Autodesk Fusion 360 part; units mm, degrees
note: some values were not read from the file. Set by a fixed rule: which sketch regions a step uses.
(part 19 of 20)
  spline S109 degree 5 poles (-22.9448, 17.8091) (-22.9448, 17.8092) (-22.945, 17.8093) (-22.9453, 17.8095) (-22.9457, 17.8098) (-22.9463, 17.8103) (-22.9469, 17.8108) (-22.9477, 17.8114) (-22.9486, 17.812) (-22.9496, 17.8127) (-22.9506, 17.8135) (-22.9518, 17.8144) (-22.953, 17.8153) (-22.9543, 17.8162) (-22.9557, 17.8172) (-22.9572, 17.8183) (-22.9588, 17.8195) (-22.9604, 17.8207) (-22.9622, 17.8219) (-22.964, 17.8232) (-22.9659, 17.8246) (-22.9679, 17.826) (-22.9699, 17.8274) (-22.9721, 17.8289) (-22.9743, 17.8305) (-22.9766, 17.8321) (-22.979, 17.8337) (-22.9814, 17.8354) (-22.984, 17.8372) (-22.9866, 17.8389) (-22.9893, 17.8408) (-22.992, 17.8427) (-22.9948, 17.8446) (-22.9978, 17.8465) (-23.0007, 17.8485) (-23.0038, 17.8506) (-23.0069, 17.8527) (-23.0101, 17.8548) (-23.0134, 17.857) (-23.0167, 17.8592) (-23.0201, 17.8614) (-23.0236, 17.8637) (-23.0271, 17.866) (-23.0308, 17.8683) (-23.0344, 17.8707) (-23.0382, 17.8731) (-23.042, 17.8756) (-23.0459, 17.8781) (-23.0499, 17.8806) (-23.0539, 17.8831) (-23.058, 17.8857) (-23.0621, 17.8883) (-23.0664, 17.891) (-23.0706, 17.8937) (-23.075, 17.8964) (-23.0794, 17.8991) (-23.0839, 17.9019) (-23.0884, 17.9047) (-23.093, 17.9075) (-23.0977, 17.9103) (-23.1024, 17.9132) (-23.1072, 17.9161) (-23.1121, 17.9191) (-23.117, 17.922) (-23.122, 17.925) (-23.127, 17.928) (-23.1321, 17.931) (-23.1373, 17.9341) (-23.1425, 17.9372) (-23.1478, 17.9403) (-23.1531, 17.9434) (-23.1585, 17.9466) (-23.164, 17.9497) (-23.1695, 17.9529) (-23.1751, 17.9562) (-23.1807, 17.9594) (-23.1864, 17.9627) (-23.1921, 17.9659) (-23.1979, 17.9692) (-23.2038, 17.9726) (-23.2097, 17.9759) (-23.2157, 17.9793) (-23.2217, 17.9826) (-23.2278, 17.986) (-23.234, 17.9895) (-23.2402, 17.9929) (-23.2464, 17.9963) (-23.2527, 17.9998) (-23.2591, 18.0033) (-23.2655, 18.0068) (-23.272, 18.0103) (-23.2785, 18.0139) (-23.2851, 18.0174) (-23.2918, 18.021) (-23.2984, 18.0246) (-23.3052, 18.0282) (-23.312, 18.0318) (-23.3188, 18.0354) (-23.3257, 18.039) (-23.3327, 18.0427) (-23.3397, 18.0464) (-23.3468, 18.0501) (-23.3539, 18.0538) (-23.361, 18.0575) (-23.3683, 18.0612) (-23.3755, 18.0649) (-23.3828, 18.0687) (-23.3902, 18.0724) (-23.3976, 18.0762) (-23.4051, 18.08) (-23.4126, 18.0838) (-23.4202, 18.0876) (-23.4278, 18.0914) (-23.4355, 18.0952) (-23.4432, 18.0991) (-23.451, 18.1029) (-23.4588, 18.1068) (-23.4666, 18.1106) (-23.4746, 18.1145) (-23.4825, 18.1184) (-23.4905, 18.1223) (-23.4986, 18.1262) (-23.5067, 18.1301) (-23.5149, 18.134) (-23.5231, 18.1379) (-23.5313, 18.1419) (-23.5396, 18.1458) (-23.548, 18.1498) (-23.5564, 18.1537) (-23.5648, 18.1577) (-23.5733, 18.1617) (-23.5818, 18.1657) (-23.5904, 18.1696) (-23.5991, 18.1736) (-23.6077, 18.1776) (-23.6165, 18.1816) (-23.6252, 18.1857) (-23.634, 18.1897) (-23.6429, 18.1937) (-23.6518, 18.1977) (-23.6607, 18.2018) (-23.6697, 18.2058) (-23.6788, 18.2098) (-23.6879, 18.2139) (-23.697, 18.2179) (-23.7062, 18.222) (-23.7154, 18.226) (-23.7247, 18.2301) (-23.734, 18.2342) (-23.7433, 18.2383) (-23.7527, 18.2423) (-23.7622, 18.2464) (-23.7716, 18.2505) (-23.7812, 18.2546) (-23.7907, 18.2587) (-23.8004, 18.2627) (-23.81, 18.2668) (-23.8197, 18.2709) (-23.8295, 18.275) (-23.8393, 18.2791) (-23.8491, 18.2832) (-23.859, 18.2873) (-23.8689, 18.2914) (-23.8788, 18.2955) (-23.8888, 18.2996) (-23.8989, 18.3038) (-23.909, 18.3079) (-23.9191, 18.312) (-23.9292, 18.3161) (-23.9395, 18.3202) (-23.9497, 18.3243) (-23.96, 18.3284) (-23.9703, 18.3325) (-23.9807, 18.3366) (-23.9911, 18.3408) (-24.0016, 18.3449) (-24.0121, 18.349) (-24.0226, 18.3531) (-24.0332, 18.3572) (-24.0438, 18.3613) (-24.0545, 18.3654) (-24.0652, 18.3695) (-24.0759, 18.3736) (-24.0867, 18.3777) (-24.0975, 18.3818) (-24.1084, 18.3859) (-24.1193, 18.39) (-24.1302, 18.3941) (-24.1412, 18.3982) (-24.1522, 18.4023) (-24.1633, 18.4064) (-24.1744, 18.4105) (-24.1855, 18.4146) (-24.1967, 18.4187) (-24.2079, 18.4228) (-24.2191, 18.4269) (-24.2304, 18.4309) (-24.2417, 18.435) (-24.2531, 18.4391) (-24.2645, 18.4431) (-24.276, 18.4472) (-24.2874, 18.4513) (-24.299, 18.4553) (-24.3105, 18.4594) (-24.3221, 18.4634) (-24.3337, 18.4675) (-24.3454, 18.4715) (-24.3571, 18.4756) (-24.3689, 18.4796) (-24.3806, 18.4836) (-24.3925, 18.4877) (-24.4043, 18.4917) (-24.4162, 18.4957) (-24.4281, 18.4997) (-24.4401, 18.5037) (-24.4521, 18.5077) (-24.4642, 18.5117) (-24.4762, 18.5157) (-24.4884, 18.5197) (-24.5005, 18.5237) (-24.5127, 18.5277) (-24.5249, 18.5316) (-24.5372, 18.5356) (-24.5495, 18.5395) (-24.5618, 18.5435) (-24.5742, 18.5475) (-24.5866, 18.5514) (-24.599, 18.5553) (-24.6115, 18.5593) (-24.624, 18.5632) (-24.6365, 18.5671) (-24.6491, 18.571) (-24.6617, 18.5749) (-24.6744, 18.5788) (-24.6871, 18.5827) (-24.6998, 18.5866) (-24.7125, 18.5905) (-24.7253, 18.5943) (-24.7382, 18.5982) (-24.751, 18.6021) (-24.7639, 18.6059) (-24.7743, 18.609) (-24.782, 18.6113) (-24.7872, 18.6128) (-24.7898, 18.6136) knots 0 0 0 0 0 0 0.00416667 0.00833333 0.0125 0.01666667 0.02083333 0.025 0.02916667 0.03333333 0.0375 0.04166667 0.04583333 0.05 0.05416667 0.05833333 0.0625 0.06666667 0.07083333 0.075 0.07916667 0.08333333 0.0875 0.09166667 0.09583333 0.1 0.10416667 0.10833333 0.1125 0.11666667 0.12083333 0.125 0.12916667 0.13333333 0.1375 0.14166667 0.14583333 0.15 0.15416667 0.15833333 0.1625 0.16666667 0.17083333 0.175 0.17916667 0.18333333 0.1875 0.19166667 0.19583333 0.2 0.20416667 0.20833333 0.2125 0.21666667 0.22083333 0.225 0.22916667 0.23333333 0.2375 0.24166667 0.24583333 0.25 0.25416667 0.25833333 0.2625 0.26666667 0.27083333 0.275 0.27916667 0.28333333 0.2875 0.29166667 0.29583333 0.3 0.30416667 0.30833333 0.3125 0.31666667 0.32083333 0.325 0.32916667 0.33333333 0.3375 0.34166667 0.34583333 0.35 0.35416667 0.35833333 0.3625 0.36666667 0.37083333 0.375 0.37916667 0.38333333 0.3875 0.39166667 0.39583333 0.4 0.40416667 0.40833333 0.4125 0.41666667 0.42083333 0.425 0.42916667 0.43333333 0.4375 0.44166667 0.44583333 0.45 0.45416667 0.45833333 0.4625 0.46666667 0.47083333 0.475 0.47916667 0.48333333 0.4875 0.49166667 0.49583333 0.5 0.50416667 0.50833333 0.5125 0.51666667 0.52083333 0.525 0.52916667 0.53333333 0.5375 0.54166667 0.54583333 0.55 0.55416667 0.55833333 0.5625 0.56666667 0.57083333 0.575 0.57916667 0.58333333 0.5875 0.59166667 0.59583333 0.6 0.60416667 0.60833333 0.6125 0.61666667 0.62083333 0.625 0.62916667 0.63333333 0.6375 0.64166667 0.64583333 0.65 0.65416667 0.65833333 0.6625 0.66666667 0.67083333 0.675 0.67916667 0.68333333 0.6875 0.69166667 0.69583333 0.7 0.70416667 0.70833333 0.7125 0.71666667 0.72083333 0.725 0.72916667 0.73333333 0.7375 0.74166667 0.74583333 0.75 0.75416667 0.75833333 0.7625 0.76666667 0.77083333 0.775 0.77916667 0.78333333 0.7875 0.79166667 0.79583333 0.8 0.80416667 0.80833333 0.8125 0.81666667 0.82083333 0.825 0.82916667 0.83333333 0.8375 0.84166667 0.84583333 0.85 0.85416667 0.85833333 0.8625 0.86666667 0.87083333 0.875 0.87916667 0.88333333 0.8875 0.89166667 0.89583333 0.9 0.90416667 0.90833333 0.9125 0.91666667 0.92083333 0.925 0.92916667 0.93333333 0.9375 0.94166667 0.94583333 0.95 0.95416667 0.95833333 0.9625 0.96666667 0.97083333 0.975 0.97916667 0.98333333 0.9875 0.99166667 0.99583333 1 1 1 1 1 1
  line L217 (-20.9569, 20.1094) -> (-20.9575, 20.11)
  line L218 (-13.7175, -25.6019) -> (-13.7171, -25.6012)
  line L219 (-10.9659, -26.8948) -> (-10.8547, -26.6221)
  arc A111 (30.4202, 5.9675) -> (30.2174, 6.9214) centre (0, 0) ccw
  arc A112 (27.918, 6.8665) -> (27.6109, 8.0125) centre (0, 0) ccw
  line L220 (-24.0278, 16.3184) -> (-24.0271, 16.318)
  spline S110 degree 5 poles (3.9508, 28.7753) (3.9508, 28.7754) (3.9508, 28.7756) (3.9509, 28.7759) (3.9509, 28.7764) (3.951, 28.7772) (3.9511, 28.778) (3.9512, 28.779) (3.9514, 28.7801) (3.9515, 28.7813) (3.9517, 28.7826) (3.9518, 28.784) (3.952, 28.7855) (3.9522, 28.7871) (3.9523, 28.7889) (3.9525, 28.7907) (3.9527, 28.7926) (3.9529, 28.7946) (3.9531, 28.7968) (3.9534, 28.799) (3.9536, 28.8013) (3.9538, 28.8037) (3.954, 28.8063) (3.9543, 28.8089) (3.9545, 28.8116) (3.9547, 28.8144) (3.955, 28.8172) (3.9552, 28.8202) (3.9555, 28.8233) (3.9557, 28.8264) (3.9559, 28.8297) (3.9562, 28.833) (3.9564, 28.8364) (3.9567, 28.8399) (3.9569, 28.8435) (3.9572, 28.8472) (3.9574, 28.8509) (3.9577, 28.8547) (3.9579, 28.8586) (3.9581, 28.8626) (3.9584, 28.8667) (3.9586, 28.8709) (3.9588, 28.8751) (3.959, 28.8794) (3.9593, 28.8838) (3.9595, 28.8882) (3.9597, 28.8928) (3.9599, 28.8974) (3.9601, 28.9021) (3.9603, 28.9068) (3.9605, 28.9117) (3.9607, 28.9166) (3.9609, 28.9215) (3.961, 28.9266) (3.9612, 28.9317) (3.9614, 28.9369) (3.9615, 28.9422) (3.9617, 28.9475) (3.9618, 28.9529) (3.962, 28.9584) (3.9621, 28.9639) (3.9622, 28.9695) (3.9623, 28.9752) (3.9624, 28.9809) (3.9625, 28.9867) (3.9626, 28.9926) (3.9627, 28.9985) (3.9627, 29.0045) (3.9628, 29.0106) (3.9629, 29.0167) (3.9629, 29.0229) (3.9629, 29.0291) (3.9629, 29.0355) (3.963, 29.0418) (3.963, 29.0483) (3.9629, 29.0548) (3.9629, 29.0613) (3.9629, 29.068) (3.9628, 29.0746) (3.9628, 29.0814) (3.9627, 29.0882) (3.9626, 29.095) (3.9626, 29.1019) (3.9625, 29.1089) (3.9623, 29.1159) (3.9622, 29.123) (3.9621, 29.1302) (3.9619, 29.1374) (3.9618, 29.1446) (3.9616, 29.1519) (3.9614, 29.1593) (3.9612, 29.1667) (3.961, 29.1742) (3.9607, 29.1817) (3.9605, 29.1893) (3.9603, 29.197) (3.96, 29.2047) (3.9597, 29.2124) (3.9594, 29.2202) (3.9591, 29.2281) (3.9588, 29.236) (3.9584, 29.2439) (3.9581, 29.2519) (3.9577, 29.26) (3.9573, 29.2681) (3.9569, 29.2763) (3.9565, 29.2845) (3.9561, 29.2927) (3.9556, 29.301) (3.9552, 29.3094) (3.9547, 29.3178) (3.9542, 29.3263) (3.9537, 29.3348) (3.9532, 29.3433) (3.9526, 29.3519) (3.9521, 29.3606) (3.9515, 29.3693) (3.9509, 29.378) (3.9503, 29.3868) (3.9497, 29.3957) (3.9491, 29.4045) (3.9484, 29.4135) (3.9478, 29.4225) (3.9471, 29.4315) (3.9464, 29.4406) (3.9457, 29.4497) (3.9449, 29.4588) (3.9442, 29.468) (3.9434, 29.4773) (3.9426, 29.4866) (3.9418, 29.4959) (3.941, 29.5053) (3.9402, 29.5147) (3.9393, 29.5242) (3.9384, 29.5337) (3.9375, 29.5433) (3.9366, 29.5529) (3.9357, 29.5625) (3.9348, 29.5722) (3.9338, 29.5819) (3.9328, 29.5917) (3.9318, 29.6015) (3.9308, 29.6113) (3.9297, 29.6212) (3.9287, 29.6312) (3.9276, 29.6411) (3.9265, 29.6512) (3.9254, 29.6612) (3.9243, 29.6713) (3.9231, 29.6814) (3.922, 29.6916) (3.9208, 29.7018) (3.9196, 29.7121) (3.9183, 29.7224) (3.9171, 29.7327) (3.9158, 29.7431) (3.9145, 29.7535) (3.9132, 29.764) (3.9119, 29.7744) (3.9106, 29.785) (3.9092, 29.7955) (3.9078, 29.8061) (3.9064, 29.8168) (3.905, 29.8274) (3.9035, 29.8382) (3.9021, 29.8489) (3.9006, 29.8597) (3.8991, 29.8705) (3.8976, 29.8814) (3.896, 29.8923) (3.8945, 29.9032) (3.8929, 29.9142) (3.8913, 29.9252) (3.8896, 29.9362) (3.888, 29.9473) (3.8863, 29.9584) (3.8846, 29.9696) (3.8829, 29.9807) (3.8812, 29.992) (3.8795, 30.0032) (3.8777, 30.0145) (3.8759, 30.0258) (3.8741, 30.0372) (3.8722, 30.0486) (3.8704, 30.06) (3.8685, 30.0714) (3.8666, 30.0829) (3.8647, 30.0944) (3.8628, 30.106) (3.8608, 30.1176) (3.8588, 30.1292) (3.8568, 30.1409) (3.8548, 30.1525) (3.8527, 30.1643) (3.8507, 30.176) (3.8486, 30.1878) (3.8464, 30.1996) (3.8443, 30.2115) (3.8422, 30.2233) (3.84, 30.2353) (3.8378, 30.2472) (3.8356, 30.2592) (3.8333, 30.2712) (3.831, 30.2832) (3.8288, 30.2953) (3.8264, 30.3074) (3.8241, 30.3195) (3.8217, 30.3317) (3.8194, 30.3439) (3.817, 30.3561) (3.8145, 30.3683) (3.8121, 30.3806) (3.8096, 30.3929) (3.8071, 30.4053) (3.8046, 30.4176) (3.8021, 30.43) (3.7995, 30.4424) (3.797, 30.4549) (3.7943, 30.4674) (3.7917, 30.4799) (3.7891, 30.4924) (3.7864, 30.505) (3.7837, 30.5176) (3.781, 30.5302) (3.7782, 30.5429) (3.7755, 30.5556) (3.7727, 30.5683) (3.7699, 30.581) (3.767, 30.5938) (3.7642, 30.6066) (3.7613, 30.6194) (3.7584, 30.6323) (3.7555, 30.6451) (3.7525, 30.658) (3.7496, 30.671) (3.7466, 30.6839) (3.7435, 30.6969) (3.7405, 30.7099) (3.7374, 30.723) (3.7343, 30.736) (3.7312, 30.7491) (3.7287, 30.7596) (3.7268, 30.7675) (3.7256, 30.7728) (3.7249, 30.7754) knots 0 0 0 0 0 0 0.00416667 0.00833333 0.0125 0.01666667 0.02083333 0.025 0.02916667 0.03333333 0.0375 0.04166667 0.04583333 0.05 0.05416667 0.05833333 0.0625 0.06666667 0.07083333 0.075 0.07916667 0.08333333 0.0875 0.09166667 0.09583333 0.1 0.10416667 0.10833333 0.1125 0.11666667 0.12083333 0.125 0.12916667 0.13333333 0.1375 0.14166667 0.14583333 0.15 0.15416667 0.15833333 0.1625 0.16666667 0.17083333 0.175 0.17916667 0.18333333 0.1875 0.19166667 0.19583333 0.2 0.20416667 0.20833333 0.2125 0.21666667 0.22083333 0.225 0.22916667 0.23333333 0.2375 0.24166667 0.24583333 0.25 0.25416667 0.25833333 0.2625 0.26666667 0.27083333 0.275 0.27916667 0.28333333 0.2875 0.29166667 0.29583333 0.3 0.30416667 0.30833333 0.3125 0.31666667 0.32083333 0.325 0.32916667 0.33333333 0.3375 0.34166667 0.34583333 0.35 0.35416667 0.35833333 0.3625 0.36666667 0.37083333 0.375 0.37916667 0.38333333 0.3875 0.39166667 0.39583333 0.4 0.40416667 0.40833333 0.4125 0.41666667 0.42083333 0.425 0.42916667 0.43333333 0.4375 0.44166667 0.44583333 0.45 0.45416667 0.45833333 0.4625 0.46666667 0.47083333 0.475 0.47916667 0.48333333 0.4875 0.49166667 0.49583333 0.5 0.50416667 0.50833333 0.5125 0.51666667 0.52083333 0.525 0.52916667 0.53333333 0.5375 0.54166667 0.54583333 0.55 0.55416667 0.55833333 0.5625 0.56666667 0.57083333 0.575 0.57916667 0.58333333 0.5875 0.59166667 0.59583333 0.6 0.60416667 0.60833333 0.6125 0.61666667 0.62083333 0.625 0.62916667 0.63333333 0.6375 0.64166667 0.64583333 0.65 0.65416667 0.65833333 0.6625 0.66666667 0.67083333 0.675 0.67916667 0.68333333 0.6875 0.69166667 0.69583333 0.7 0.70416667 0.70833333 0.7125 0.71666667 0.72083333 0.725 0.72916667 0.73333333 0.7375 0.74166667 0.74583333 0.75 0.75416667 0.75833333 0.7625 0.76666667 0.77083333 0.775 0.77916667 0.78333333 0.7875 0.79166667 0.79583333 0.8 0.80416667 0.80833333 0.8125 0.81666667 0.82083333 0.825 0.82916667 0.83333333 0.8375 0.84166667 0.84583333 0.85 0.85416667 0.85833333 0.8625 0.86666667 0.87083333 0.875 0.87916667 0.88333333 0.8875 0.89166667 0.89583333 0.9 0.90416667 0.90833333 0.9125 0.91666667 0.92083333 0.925 0.92916667 0.93333333 0.9375 0.94166667 0.94583333 0.95 0.95416667 0.95833333 0.9625 0.96666667 0.97083333 0.975 0.97916667 0.98333333 0.9875 0.99166667 0.99583333 1 1 1 1 1 1
  arc A113 (3.7249, 30.7754) -> (2.755, 30.8773) centre (0, 0) ccw
  circle A114 centre (0, 10) radius 1.7
  spline S111 degree 5 poles (-27.0873, 15.0758) (-27.0855, 15.0737) (-27.082, 15.0696) (-27.0767, 15.0635) (-27.0697, 15.0553) (-27.061, 15.045) (-27.0522, 15.0349) (-27.0435, 15.0247) (-27.0347, 15.0146) (-27.026, 15.0045) (-27.0173, 14.9945) (-27.0086, 14.9845) (-26.9999, 14.9745) (-26.9912, 14.9646) (-26.9825, 14.9547) (-26.9738, 14.9448) (-26.9651, 14.935) (-26.9565, 14.9252) (-26.9478, 14.9154) (-26.9392, 14.9057) (-26.9305, 14.896) (-26.9219, 14.8863) (-26.9133, 14.8767) (-26.9047, 14.8671) (-26.8961, 14.8576) (-26.8875, 14.8481) (-26.8789, 14.8386) (-26.8703, 14.8291) (-26.8618, 14.8197) (-26.8532, 14.8104) (-26.8447, 14.801) (-26.8361, 14.7917) (-26.8276, 14.7824) (-26.8191, 14.7732) (-26.8106, 14.764) (-26.8021, 14.7549) (-26.7937, 14.7457) (-26.7852, 14.7366) (-26.7767, 14.7276) (-26.7683, 14.7186) (-26.7599, 14.7096) (-26.7515, 14.7006) (-26.7431, 14.6917) (-26.7347, 14.6829) (-26.7263, 14.674) (-26.7179, 14.6652) (-26.7096, 14.6565) (-26.7012, 14.6477) (-26.6929, 14.639) (-26.6846, 14.6304) (-26.6763, 14.6218) (-26.668, 14.6132) (-26.6597, 14.6046) (-26.6514, 14.5961) (-26.6432, 14.5877) (-26.635, 14.5792) (-26.6267, 14.5708) (-26.6185, 14.5625) (-26.6103, 14.5541) (-26.6022, 14.5459) (-26.594, 14.5376) (-26.5858, 14.5294) (-26.5777, 14.5212) (-26.5696, 14.5131) (-26.5615, 14.505) (-26.5534, 14.4969) (-26.5453, 14.4889) (-26.5373, 14.4809) (-26.5292, 14.4729) (-26.5212, 14.465) (-26.5132, 14.4571) (-26.5052, 14.4493) (-26.4972, 14.4415) (-26.4893, 14.4337) (-26.4813, 14.426) (-26.4734, 14.4183) (-26.4655, 14.4106) (-26.4576, 14.403) (-26.4497, 14.3954) (-26.4419, 14.3879) (-26.434, 14.3804) (-26.4262, 14.3729) (-26.4184, 14.3655) (-26.4106, 14.3581) (-26.4029, 14.3508) (-26.3951, 14.3435) (-26.3874, 14.3362) (-26.3797, 14.3289) (-26.372, 14.3217) (-26.3643, 14.3146) (-26.3567, 14.3075) (-26.3491, 14.3004) (-26.3414, 14.2933) (-26.3339, 14.2863) (-26.3263, 14.2794) (-26.3188, 14.2724) (-26.3112, 14.2656) (-26.3037, 14.2587) (-26.2962, 14.2519) (-26.2888, 14.2451) (-26.2813, 14.2384) (-26.2739, 14.2317) (-26.2665, 14.225) (-26.2592, 14.2184) (-26.2518, 14.2119) (-26.2445, 14.2053) (-26.2372, 14.1988) (-26.2299, 14.1924) (-26.2227, 14.1859) (-26.2154, 14.1796) (-26.2082, 14.1732) (-26.201, 14.1669) (-26.1939, 14.1607) (-26.1868, 14.1544) (-26.1796, 14.1483) (-26.1726, 14.1421) (-26.1655, 14.136) (-26.1585, 14.13) (-26.1515, 14.1239) (-26.1445, 14.118) (-26.1375, 14.112) (-26.1306, 14.1061) (-26.1237, 14.1003) (-26.1168, 14.0945) (-26.11, 14.0887) (-26.1032, 14.0829) (-26.0964, 14.0772) (-26.0896, 14.0716) (-26.0829, 14.066) (-26.0762, 14.0604) (-26.0695, 14.0549) (-26.0629, 14.0494) (-26.0563, 14.0439) (-26.0497, 14.0385) (-26.0431, 14.0332) (-26.0366, 14.0278) (-26.0301, 14.0225) (-26.0236, 14.0173) (-26.0172, 14.0121) (-26.0108, 14.0069) (-26.0044, 14.0018) (-25.9981, 13.9967) (-25.9918, 13.9917) (-25.9855, 13.9867) (-25.9793, 13.9818) (-25.9731, 13.9769) (-25.9669, 13.972) (-25.9608, 13.9672) (-25.9547, 13.9624) (-25.9486, 13.9576) (-25.9426, 13.9529) (-25.9366, 13.9483) (-25.9306, 13.9437) (-25.9247, 13.9391) (-25.9188, 13.9346) (-25.913, 13.9301) (-25.9072, 13.9257) (-25.9014, 13.9213) (-25.8957, 13.9169) (-25.89, 13.9126) (-25.8843, 13.9083) (-25.8787, 13.9041) (-25.8731, 13.8999) (-25.8676, 13.8958) (-25.8621, 13.8917) (-25.8566, 13.8876) (-25.8512, 13.8836) (-25.8458, 13.8797) (-25.8405, 13.8758) (-25.8352, 13.8719) (-25.8299, 13.8681) (-25.8247, 13.8643) (-25.8195, 13.8605) (-25.8144, 13.8568) (-25.8093, 13.8532) (-25.8043, 13.8496) (-25.7993, 13.846) (-25.7944, 13.8425) (-25.7895, 13.839) (-25.7847, 13.8356) (-25.7799, 13.8322) (-25.7751, 13.8289) (-25.7704, 13.8256) (-25.7658, 13.8224) (-25.7612, 13.8192) (-25.7566, 13.816) (-25.7521, 13.8129) (-25.7476, 13.8098) (-25.7432, 13.8068) (-25.7389, 13.8039) (-25.7346, 13.8009) (-25.7304, 13.7981) (-25.7262, 13.7952) (-25.722, 13.7925) (-25.718, 13.7897) (-25.7139, 13.787) (-25.71, 13.7844) (-25.706, 13.7818) (-25.7022, 13.7793) (-25.6984, 13.7768) (-25.6947, 13.7743) (-25.691, 13.7719) (-25.6874, 13.7696) (-25.6838, 13.7673) (-25.6803, 13.765) (-25.6769, 13.7628) (-25.6735, 13.7607) (-25.6702, 13.7586) (-25.667, 13.7565) (-25.6638, 13.7545) (-25.6607, 13.7526) (-25.6577, 13.7506) (-25.6547, 13.7488) (-25.6518, 13.747) (-25.6489, 13.7452) (-25.6462, 13.7435) (-25.6435, 13.7419) (-25.6409, 13.7403) (-25.6383, 13.7387) (-25.6358, 13.7372) (-25.6334, 13.7358) (-25.6311, 13.7344) (-25.6289, 13.733) (-25.6267, 13.7317) (-25.6246, 13.7305) (-25.6226, 13.7293) (-25.6207, 13.7282) (-25.6188, 13.7271) (-25.6171, 13.7261) (-25.6154, 13.7251) (-25.6138, 13.7242) (-25.6123, 13.7233) (-25.6109, 13.7225) (-25.6096, 13.7217) (-25.6083, 13.721) (-25.6072, 13.7204) (-25.6061, 13.7198) (-25.6052, 13.7193) (-25.6043, 13.7188) (-25.6036, 13.7184) (-25.6029, 13.718) (-25.6025, 13.7178) (-25.6022, 13.7176) (-25.602, 13.7175) (-25.6019, 13.7175) knots -1 -1 -1 -1 -1 -1 -0.99583333 -0.99166667 -0.9875 -0.98333333 -0.97916667 -0.975 -0.97083333 -0.96666667 -0.9625 -0.95833333 -0.95416667 -0.95 -0.94583333 -0.94166667 -0.9375 -0.93333333 -0.92916667 -0.925 -0.92083333 -0.91666667 -0.9125 -0.90833333 -0.90416667 -0.9 -0.89583333 -0.89166667 -0.8875 -0.88333333 -0.87916667 -0.875 -0.87083333 -0.86666667 -0.8625 -0.85833333 -0.85416667 -0.85 -0.84583333 -0.84166667 -0.8375 -0.83333333 -0.82916667 -0.825 -0.82083333 -0.81666667 -0.8125 -0.80833333 -0.80416667 -0.8 -0.79583333 -0.79166667 -0.7875 -0.78333333 -0.77916667 -0.775 -0.77083333 -0.76666667 -0.7625 -0.75833333 -0.75416667 -0.75 -0.74583333 -0.74166667 -0.7375 -0.73333333 -0.72916667 -0.725 -0.72083333 -0.71666667 -0.7125 -0.70833333 -0.70416667 -0.7 -0.69583333 -0.69166667 -0.6875 -0.68333333 -0.67916667 -0.675 -0.67083333 -0.66666667 -0.6625 -0.65833333 -0.65416667 -0.65 -0.64583333 -0.64166667 -0.6375 -0.63333333 -0.62916667 -0.625 -0.62083333 -0.61666667 -0.6125 -0.60833333 -0.60416667 -0.6 -0.59583333 -0.59166667 -0.5875 -0.58333333 -0.57916667 -0.575 -0.57083333 -0.56666667 -0.5625 -0.55833333 -0.55416667 -0.55 -0.54583333 -0.54166667 -0.5375 -0.53333333 -0.52916667 -0.525 -0.52083333 -0.51666667 -0.5125 -0.50833333 -0.50416667 -0.5 -0.49583333 -0.49166667 -0.4875 -0.48333333 -0.47916667 -0.475 -0.47083333 -0.46666667 -0.4625 -0.45833333 -0.45416667 -0.45 -0.44583333 -0.44166667 -0.4375 -0.43333333 -0.42916667 -0.425 -0.42083333 -0.41666667 -0.4125 -0.40833333 -0.40416667 -0.4 -0.39583333 -0.39166667 -0.3875 -0.38333333 -0.37916667 -0.375 -0.37083333 -0.36666667 -0.3625 -0.35833333 -0.35416667 -0.35 -0.34583333 -0.34166667 -0.3375 -0.33333333 -0.32916667 -0.325 -0.32083333 -0.31666667 -0.3125 -0.30833333 -0.30416667 -0.3 -0.29583333 -0.29166667 -0.2875 -0.28333333 -0.27916667 -0.275 -0.27083333 -0.26666667 -0.2625 -0.25833333 -0.25416667 -0.25 -0.24583333 -0.24166667 -0.2375 -0.23333333 -0.22916667 -0.225 -0.22083333 -0.21666667 -0.2125 -0.20833333 -0.20416667 -0.2 -0.19583333 -0.19166667 -0.1875 -0.18333333 -0.17916667 -0.175 -0.17083333 -0.16666667 -0.1625 -0.15833333 -0.15416667 -0.15 -0.14583333 -0.14166667 -0.1375 -0.13333333 -0.12916667 -0.125 -0.12083333 -0.11666667 -0.1125 -0.10833333 -0.10416667 -0.1 -0.09583333 -0.09166667 -0.0875 -0.08333333 -0.07916667 -0.075 -0.07083333 -0.06666667 -0.0625 -0.05833333 -0.05416667 -0.05 -0.04583333 -0.04166667 -0.0375 -0.03333333 -0.02916667 -0.025 -0.02083333 -0.01666667 -0.0125 -0.00833333 -0.00416667 0 0 0 0 0 0
  circle A115 centre (-10, 0) radius 1.7
  line L221 (2.1183, 28.9679) -> (2.1182, 28.9671)
  line L222 (-24.4297, 15.1575) -> (-24.6799, 15.3128)
  line L223 (2.1182, 28.9671) -> (2.0967, 28.6734)
  arc A116 (-25.3417, 13.578) -> (-25.8803, 12.5209) centre (0, 0) ccw
  spline S112 degree 5 poles (-25.363, 17.8246) (-25.3615, 17.8224) (-25.3584, 17.8179) (-25.3539, 17.8112) (-25.3477, 17.8023) (-25.3401, 17.7913) (-25.3325, 17.7802) (-25.3248, 17.7692) (-25.3172, 17.7583) (-25.3096, 17.7473) (-25.3019, 17.7364) (-25.2943, 17.7256) (-25.2867, 17.7147) (-25.2791, 17.7039) (-25.2715, 17.6932) (-25.2639, 17.6825) (-25.2563, 17.6718) (-25.2487, 17.6611) (-25.2411, 17.6505) (-25.2335, 17.6399) (-25.2259, 17.6294) (-25.2184, 17.6189) (-25.2108, 17.6084) (-25.2032, 17.598) (-25.1957, 17.5876) (-25.1881, 17.5772) (-25.1806, 17.5669) (-25.1731, 17.5566) (-25.1655, 17.5464) (-25.158, 17.5361) (-25.1505, 17.526) (-25.143, 17.5158) (-25.1355, 17.5057) (-25.128, 17.4956) (-25.1205, 17.4856) (-25.113, 17.4756) (-25.1055, 17.4657) (-25.0981, 17.4557) (-25.0906, 17.4458) (-25.0832, 17.436) (-25.0757, 17.4262) (-25.0683, 17.4164) (-25.0609, 17.4067) (-25.0534, 17.397) (-25.046, 17.3873) (-25.0386, 17.3777) (-25.0312, 17.3681) (-25.0238, 17.3585) (-25.0165, 17.349) (-25.0091, 17.3395) (-25.0017, 17.3301) (-24.9944, 17.3207) (-24.9871, 17.3113) (-24.9797, 17.302) (-24.9724, 17.2927) (-24.9651, 17.2835) (-24.9578, 17.2743) (-24.9505, 17.2651) (-24.9432, 17.2559) (-24.936, 17.2469) (-24.9287, 17.2378) (-24.9215, 17.2288) (-24.9142, 17.2198) (-24.907, 17.2108) (-24.8998, 17.2019) (-24.8926, 17.1931) (-24.8854, 17.1842) (-24.8782, 17.1754) (-24.8711, 17.1667) (-24.8639, 17.158) (-24.8568, 17.1493) (-24.8496, 17.1407) (-24.8425, 17.1321) (-24.8354, 17.1235) (-24.8283, 17.115) (-24.8212, 17.1065) (-24.8142, 17.0981) (-24.8071, 17.0897) (-24.8001, 17.0813) (-24.7931, 17.073) (-24.7861, 17.0647) (-24.7791, 17.0565) (-24.7721, 17.0483) (-24.7651, 17.0401) (-24.7582, 17.032) (-24.7512, 17.0239) (-24.7443, 17.0159) (-24.7374, 17.0079) (-24.7305, 16.9999) (-24.7236, 16.992) (-24.7168, 16.9841) (-24.7099, 16.9763) (-24.7031, 16.9685) (-24.6963, 16.9607) (-24.6895, 16.953) (-24.6827, 16.9453) (-24.6759, 16.9377) (-24.6692, 16.9301) (-24.6625, 16.9225) (-24.6558, 16.915) (-24.6491, 16.9075) (-24.6424, 16.9001) (-24.6357, 16.8927) (-24.6291, 16.8854) (-24.6225, 16.8781) (-24.6159, 16.8708) (-24.6093, 16.8636) (-24.6027, 16.8564) (-24.5962, 16.8492) (-24.5897, 16.8421) (-24.5831, 16.8351) (-24.5767, 16.8281) (-24.5702, 16.8211) (-24.5638, 16.8142) (-24.5573, 16.8073) (-24.5509, 16.8004) (-24.5446, 16.7936) (-24.5382, 16.7869) (-24.5319, 16.7801) (-24.5255, 16.7735) (-24.5192, 16.7668) (-24.513, 16.7602) (-24.5067, 16.7537) (-24.5005, 16.7472) (-24.4943, 16.7407) (-24.4881, 16.7343) (-24.482, 16.7279) (-24.4758, 16.7216) (-24.4697, 16.7153) (-24.4636, 16.7091) (-24.4576, 16.7029) (-24.4515, 16.6967) (-24.4455, 16.6906) (-24.4395, 16.6845) (-24.4336, 16.6785) (-24.4277, 16.6725) (-24.4218, 16.6666) (-24.4159, 16.6607) (-24.41, 16.6549) (-24.4042, 16.6491) (-24.3984, 16.6433) (-24.3926, 16.6376) (-24.3869, 16.6319) (-24.3812, 16.6263) (-24.3755, 16.6207) (-24.3698, 16.6152) (-24.3642, 16.6097) (-24.3586, 16.6043) (-24.353, 16.5989) (-24.3475, 16.5935) (-24.342, 16.5882) (-24.3365, 16.583) (-24.3311, 16.5778) (-24.3257, 16.5726) (-24.3203, 16.5675) (-24.3149, 16.5624) (-24.3096, 16.5574) (-24.3043, 16.5524) (-24.2991, 16.5475) (-24.2939, 16.5426) (-24.2887, 16.5378) (-24.2835, 16.533) (-24.2784, 16.5282) (-24.2733, 16.5236) (-24.2683, 16.5189) (-24.2633, 16.5143) (-24.2583, 16.5098) (-24.2534, 16.5053) (-24.2485, 16.5008) (-24.2436, 16.4964) (-24.2388, 16.492) (-24.234, 16.4877) (-24.2293, 16.4835) (-24.2246, 16.4793) (-24.2199, 16.4751) (-24.2153, 16.471) (-24.2107, 16.4669) (-24.2062, 16.4629) (-24.2017, 16.459) (-24.1972, 16.455) (-24.1928, 16.4512) (-24.1884, 16.4474) (-24.1841, 16.4436) (-24.1798, 16.4399) (-24.1755, 16.4362) (-24.1713, 16.4326) (-24.1672, 16.4291) (-24.1631, 16.4256) (-24.159, 16.4221) (-24.155, 16.4187) (-24.151, 16.4153) (-24.1471, 16.412) (-24.1432, 16.4088) (-24.1394, 16.4056) (-24.1356, 16.4024) (-24.1319, 16.3994) (-24.1283, 16.3963) (-24.1246, 16.3933) (-24.1211, 16.3904) (-24.1176, 16.3875) (-24.1141, 16.3847) (-24.1107, 16.3819) (-24.1073, 16.3792) (-24.104, 16.3766) (-24.1008, 16.374) (-24.0976, 16.3714) (-24.0945, 16.3689) (-24.0914, 16.3665) (-24.0884, 16.3641) (-24.0855, 16.3618) (-24.0826, 16.3595) (-24.0798, 16.3573) (-24.077, 16.3551) (-24.0743, 16.353) (-24.0717, 16.351) (-24.0691, 16.349) (-24.0666, 16.3471) (-24.0641, 16.3452) (-24.0618, 16.3434) (-24.0595, 16.3416) (-24.0572, 16.3399) (-24.0551, 16.3383) (-24.053, 16.3367) (-24.051, 16.3352) (-24.049, 16.3338) (-24.0471, 16.3324) (-24.0453, 16.331) (-24.0436, 16.3298) (-24.042, 16.3286) (-24.0404, 16.3274) (-24.0389, 16.3263) (-24.0375, 16.3253) (-24.0362, 16.3244) (-24.035, 16.3235) (-24.0338, 16.3227) (-24.0327, 16.3219) (-24.0317, 16.3212) (-24.0309, 16.3206) (-24.0301, 16.32) (-24.0294, 16.3195) (-24.0287, 16.3191) (-24.0283, 16.3188) (-24.0281, 16.3186) (-24.0279, 16.3185) (-24.0278, 16.3184) knots -1 -1 -1 -1 -1 -1 -0.99583333 -0.99166667 -0.9875 -0.98333333 -0.97916667 -0.975 -0.97083333 -0.96666667 -0.9625 -0.95833333 -0.95416667 -0.95 -0.94583333 -0.94166667 -0.9375 -0.93333333 -0.92916667 -0.925 -0.92083333 -0.91666667 -0.9125 -0.90833333 -0.90416667 -0.9 -0.89583333 -0.89166667 -0.8875 -0.88333333 -0.87916667 -0.875 -0.87083333 -0.86666667 -0.8625 -0.85833333 -0.85416667 -0.85 -0.84583333 -0.84166667 -0.8375 -0.83333333 -0.82916667 -0.825 -0.82083333 -0.81666667 -0.8125 -0.80833333 -0.80416667 -0.8 -0.79583333 -0.79166667 -0.7875 -0.78333333 -0.77916667 -0.775 -0.77083333 -0.76666667 -0.7625 -0.75833333 -0.75416667 -0.75 -0.74583333 -0.74166667 -0.7375 -0.73333333 -0.72916667 -0.725 -0.72083333 -0.71666667 -0.7125 -0.70833333 -0.70416667 -0.7 -0.69583333 -0.69166667 -0.6875 -0.68333333 -0.67916667 -0.675 -0.67083333 -0.66666667 -0.6625 -0.65833333 -0.65416667 -0.65 -0.64583333 -0.64166667 -0.6375 -0.63333333 -0.62916667 -0.625 -0.62083333 -0.61666667 -0.6125 -0.60833333 -0.60416667 -0.6 -0.59583333 -0.59166667 -0.5875 -0.58333333 -0.57916667 -0.575 -0.57083333 -0.56666667 -0.5625 -0.55833333 -0.55416667 -0.55 -0.54583333 -0.54166667 -0.5375 -0.53333333 -0.52916667 -0.525 -0.52083333 -0.51666667 -0.5125 -0.50833333 -0.50416667 -0.5 -0.49583333 -0.49166667 -0.4875 -0.48333333 -0.47916667 -0.475 -0.47083333 -0.46666667 -0.4625 -0.45833333 -0.45416667 -0.45 -0.44583333 -0.44166667 -0.4375 -0.43333333 -0.42916667 -0.425 -0.42083333 -0.41666667 -0.4125 -0.40833333 -0.40416667 -0.4 -0.39583333 -0.39166667 -0.3875 -0.38333333 -0.37916667 -0.375 -0.37083333 -0.36666667 -0.3625 -0.35833333 -0.35416667 -0.35 -0.34583333 -0.34166667 -0.3375 -0.33333333 -0.32916667 -0.325 -0.32083333 -0.31666667 -0.3125 -0.30833333 -0.30416667 -0.3 -0.29583333 -0.29166667 -0.2875 -0.28333333 -0.27916667 -0.275 -0.27083333 -0.26666667 -0.2625 -0.25833333 -0.25416667 -0.25 -0.24583333 -0.24166667 -0.2375 -0.23333333 -0.22916667 -0.225 -0.22083333 -0.21666667 -0.2125 -0.20833333 -0.20416667 -0.2 -0.19583333 -0.19166667 -0.1875 -0.18333333 -0.17916667 -0.175 -0.17083333 -0.16666667 -0.1625 -0.15833333 -0.15416667 -0.15 -0.14583333 -0.14166667 -0.1375 -0.13333333 -0.12916667 -0.125 -0.12083333 -0.11666667 -0.1125 -0.10833333 -0.10416667 -0.1 -0.09583333 -0.09166667 -0.0875 -0.08333333 -0.07916667 -0.075 -0.07083333 -0.06666667 -0.0625 -0.05833333 -0.05416667 -0.05 -0.04583333 -0.04166667 -0.0375 -0.03333333 -0.02916667 -0.025 -0.02083333 -0.01666667 -0.0125 -0.00833333 -0.00416667 0 0 0 0 0 0
  spline S113 degree 5 poles (-24.6806, 15.3132) (-24.6807, 15.3132) (-24.6809, 15.3133) (-24.6812, 15.3135) (-24.6816, 15.3138) (-24.6822, 15.3142) (-24.683, 15.3146) (-24.6838, 15.3151) (-24.6848, 15.3157) (-24.6858, 15.3163) (-24.6869, 15.3169) (-24.6881, 15.3177) (-24.6895, 15.3184) (-24.6909, 15.3193) (-24.6924, 15.3201) (-24.694, 15.321) (-24.6956, 15.322) (-24.6974, 15.323) (-24.6993, 15.3241) (-24.7012, 15.3252) (-24.7033, 15.3263) (-24.7054, 15.3275) (-24.7076, 15.3287) (-24.7099, 15.33) (-24.7122, 15.3313) (-24.7147, 15.3327) (-24.7172, 15.3341) (-24.7198, 15.3355) (-24.7225, 15.337) (-24.7253, 15.3385) (-24.7282, 15.34) (-24.7311, 15.3416) (-24.7341, 15.3432) (-24.7372, 15.3449) (-24.7404, 15.3465) (-24.7437, 15.3482) (-24.747, 15.35) (-24.7504, 15.3518) (-24.7539, 15.3536) (-24.7574, 15.3554) (-24.761, 15.3573) (-24.7647, 15.3592) (-24.7685, 15.3611) (-24.7723, 15.3631) (-24.7763, 15.3651) (-24.7802, 15.3671) (-24.7843, 15.3691) (-24.7884, 15.3712) (-24.7926, 15.3733) (-24.7969, 15.3754) (-24.8012, 15.3775) (-24.8056, 15.3797) (-24.8101, 15.3819) (-24.8147, 15.3841) (-24.8193, 15.3863) (-24.8239, 15.3886) (-24.8287, 15.3909) (-24.8335, 15.3932) (-24.8384, 15.3955) (-24.8433, 15.3979) (-24.8483, 15.4002) (-24.8534, 15.4026) (-24.8585, 15.405) (-24.8637, 15.4075) (-24.869, 15.4099) (-24.8743, 15.4124) (-24.8797, 15.4149) (-24.8852, 15.4174) (-24.8907, 15.4199) (-24.8962, 15.4224) (-24.9019, 15.425) (-24.9076, 15.4275) (-24.9133, 15.4301) (-24.9192, 15.4327) (-24.925, 15.4353) (-24.931, 15.438) (-24.937, 15.4406) (-24.943, 15.4433) (-24.9492, 15.446) (-24.9553, 15.4486) (-24.9616, 15.4514) (-24.9679, 15.4541) (-24.9742, 15.4568) (-24.9806, 15.4595) (-24.9871, 15.4623) (-24.9936, 15.4651) (-25.0002, 15.4678) (-25.0069, 15.4706) (-25.0136, 15.4734) (-25.0203, 15.4762) (-25.0271, 15.4791) (-25.034, 15.4819) (-25.0409, 15.4848) (-25.0479, 15.4876) (-25.0549, 15.4905) (-25.062, 15.4933) (-25.0691, 15.4962) (-25.0763, 15.4991) (-25.0836, 15.502) (-25.0909, 15.5049) (-25.0982, 15.5078) (-25.1056, 15.5108) (-25.1131, 15.5137) (-25.1206, 15.5166) (-25.1282, 15.5196) (-25.1358, 15.5226) (-25.1434, 15.5255) (-25.1512, 15.5285) (-25.1589, 15.5315) (-25.1668, 15.5344) (-25.1746, 15.5374) (-25.1826, 15.5404) (-25.1905, 15.5434) (-25.1986, 15.5464) (-25.2066, 15.5494) (-25.2148, 15.5524) (-25.2229, 15.5555) (-25.2312, 15.5585) (-25.2394, 15.5615) (-25.2478, 15.5645) (-25.2562, 15.5676) (-25.2646, 15.5706) (-25.2731, 15.5737) (-25.2816, 15.5767) (-25.2901, 15.5798) (-25.2988, 15.5828) (-25.3074, 15.5859) (-25.3161, 15.5889) (-25.3249, 15.592) (-25.3337, 15.595) (-25.3426, 15.5981) (-25.3515, 15.6012) (-25.3604, 15.6042) (-25.3694, 15.6073) (-25.3785, 15.6104) (-25.3876, 15.6134) (-25.3967, 15.6165) (-25.4059, 15.6196) (-25.4151, 15.6227) (-25.4244, 15.6257) (-25.4337, 15.6288) (-25.4431, 15.6319) (-25.4525, 15.635) (-25.462, 15.638) (-25.4715, 15.6411) (-25.481, 15.6442) (-25.4906, 15.6473) (-25.5003, 15.6503) (-25.5099, 15.6534) (-25.5197, 15.6565) (-25.5294, 15.6596) (-25.5393, 15.6626) (-25.5491, 15.6657) (-25.559, 15.6688) (-25.569, 15.6718) (-25.579, 15.6749) (-25.589, 15.6779) (-25.5991, 15.681) (-25.6092, 15.6841) (-25.6194, 15.6871) (-25.6296, 15.6902) (-25.6398, 15.6932) (-25.6501, 15.6963) (-25.6604, 15.6993) (-25.6708, 15.7023) (-25.6812, 15.7054) (-25.6917, 15.7084) (-25.7022, 15.7114) (-25.7127, 15.7145) (-25.7233, 15.7175) (-25.7339, 15.7205) (-25.7446, 15.7235) (-25.7553, 15.7265) (-25.766, 15.7295) (-25.7768, 15.7325) (-25.7877, 15.7355) (-25.7985, 15.7385) (-25.8094, 15.7415) (-25.8204, 15.7445) (-25.8314, 15.7475) (-25.8424, 15.7504) (-25.8535, 15.7534) (-25.8646, 15.7564) (-25.8757, 15.7593) (-25.8869, 15.7623) (-25.8982, 15.7652) (-25.9094, 15.7682) (-25.9207, 15.7711) (-25.9321, 15.774) (-25.9435, 15.7769) (-25.9549, 15.7798) (-25.9663, 15.7828) (-25.9778, 15.7857) (-25.9894, 15.7886) (-26.001, 15.7914) (-26.0126, 15.7943) (-26.0242, 15.7972) (-26.0359, 15.8001) (-26.0477, 15.8029) (-26.0594, 15.8058) (-26.0712, 15.8086) (-26.0831, 15.8115) (-26.095, 15.8143) (-26.1069, 15.8171) (-26.1188, 15.8199) (-26.1308, 15.8227) (-26.1428, 15.8255) (-26.1549, 15.8283) (-26.167, 15.8311) (-26.1792, 15.8339) (-26.1913, 15.8367) (-26.2035, 15.8394) (-26.2158, 15.8422) (-26.2281, 15.8449) (-26.2404, 15.8477) (-26.2528, 15.8504) (-26.2651, 15.8531) (-26.2776, 15.8558) (-26.29, 15.8585) (-26.3025, 15.8612) (-26.3151, 15.8639) (-26.3276, 15.8666) (-26.3403, 15.8692) (-26.3529, 15.8719) (-26.3656, 15.8745) (-26.3783, 15.8771) (-26.391, 15.8798) (-26.4038, 15.8824) (-26.4166, 15.885) (-26.4295, 15.8876) (-26.4424, 15.8902) (-26.4553, 15.8927) (-26.4682, 15.8953) (-26.4812, 15.8979) (-26.4943, 15.9004) (-26.5073, 15.9029) (-26.5204, 15.9055) (-26.5335, 15.908) (-26.5467, 15.9105) (-26.5599, 15.913) (-26.5731, 15.9154) (-26.5837, 15.9174) (-26.5917, 15.9189) (-26.597, 15.9199) (-26.5997, 15.9204) knots 0 0 0 0 0 0 0.00416667 0.00833333 0.0125 0.01666667 0.02083333 0.025 0.02916667 0.03333333 0.0375 0.04166667 0.04583333 0.05 0.05416667 0.05833333 0.0625 0.06666667 0.07083333 0.075 0.07916667 0.08333333 0.0875 0.09166667 0.09583333 0.1 0.10416667 0.10833333 0.1125 0.11666667 0.12083333 0.125 0.12916667 0.13333333 0.1375 0.14166667 0.14583333 0.15 0.15416667 0.15833333 0.1625 0.16666667 0.17083333 0.175 0.17916667 0.18333333 0.1875 0.19166667 0.19583333 0.2 0.20416667 0.20833333 0.2125 0.21666667 0.22083333 0.225 0.22916667 0.23333333 0.2375 0.24166667 0.24583333 0.25 0.25416667 0.25833333 0.2625 0.26666667 0.27083333 0.275 0.27916667 0.28333333 0.2875 0.29166667 0.29583333 0.3 0.30416667 0.30833333 0.3125 0.31666667 0.32083333 0.325 0.32916667 0.33333333 0.3375 0.34166667 0.34583333 0.35 0.35416667 0.35833333 0.3625 0.36666667 0.37083333 0.375 0.37916667 0.38333333 0.3875 0.39166667 0.39583333 0.4 0.40416667 0.40833333 0.4125 0.41666667 0.42083333 0.425 0.42916667 0.43333333 0.4375 0.44166667 0.44583333 0.45 0.45416667 0.45833333 0.4625 0.46666667 0.47083333 0.475 0.47916667 0.48333333 0.4875 0.49166667 0.49583333 0.5 0.50416667 0.50833333 0.5125 0.51666667 0.52083333 0.525 0.52916667 0.53333333 0.5375 0.54166667 0.54583333 0.55 0.55416667 0.55833333 0.5625 0.56666667 0.57083333 0.575 0.57916667 0.58333333 0.5875 0.59166667 0.59583333 0.6 0.60416667 0.60833333 0.6125 0.61666667 0.62083333 0.625 0.62916667 0.63333333 0.6375 0.64166667 0.64583333 0.65 0.65416667 0.65833333 0.6625 0.66666667 0.67083333 0.675 0.67916667 0.68333333 0.6875 0.69166667 0.69583333 0.7 0.70416667 0.70833333 0.7125 0.71666667 0.72083333 0.725 0.72916667 0.73333333 0.7375 0.74166667 0.74583333 0.75 0.75416667 0.75833333 0.7625 0.76666667 0.77083333 0.775 0.77916667 0.78333333 0.7875 0.79166667 0.79583333 0.8 0.80416667 0.80833333 0.8125 0.81666667 0.82083333 0.825 0.82916667 0.83333333 0.8375 0.84166667 0.84583333 0.85 0.85416667 0.85833333 0.8625 0.86666667 0.87083333 0.875 0.87916667 0.88333333 0.8875 0.89166667 0.89583333 0.9 0.90416667 0.90833333 0.9125 0.91666667 0.92083333 0.925 0.92916667 0.93333333 0.9375 0.94166667 0.94583333 0.95 0.95416667 0.95833333 0.9625 0.96666667 0.97083333 0.975 0.97916667 0.98333333 0.9875 0.99166667 0.99583333 1 1 1 1 1 1
  line L224 (-25.6012, 13.7171) -> (-25.3417, 13.578)
  arc A117 (-23.7836, 16.1526) -> (-24.4297, 15.1575) centre (0, 0) ccw
  spline S114 degree 5 poles (2.755, 30.8773) (2.7539, 30.8749) (2.7515, 30.87) (2.748, 30.8627) (2.7434, 30.853) (2.7376, 30.8408) (2.7319, 30.8287) (2.7262, 30.8165) (2.7205, 30.8044) (2.7149, 30.7924) (2.7092, 30.7803) (2.7036, 30.7683) (2.6981, 30.7563) (2.6925, 30.7443) (2.687, 30.7323) (2.6815, 30.7204) (2.6761, 30.7085) (2.6707, 30.6966) (2.6653, 30.6847) (2.6599, 30.6728) (2.6545, 30.661) (2.6492, 30.6492) (2.6439, 30.6374) (2.6387, 30.6256) (2.6335, 30.6139) (2.6283, 30.6022) (2.6231, 30.5905) (2.6179, 30.5788) (2.6128, 30.5672) (2.6077, 30.5555) (2.6027, 30.5439) (2.5977, 30.5324) (2.5927, 30.5208) (2.5877, 30.5093) (2.5827, 30.4978) (2.5778, 30.4863) (2.5729, 30.4749) (2.5681, 30.4634) (2.5632, 30.452) (2.5584, 30.4407) (2.5537, 30.4293) (2.5489, 30.418) (2.5442, 30.4067) (2.5395, 30.3954) (2.5348, 30.3841) (2.5302, 30.3729) (2.5256, 30.3617) (2.521, 30.3506) (2.5165, 30.3394) (2.5119, 30.3283) (2.5074, 30.3172) (2.503, 30.3061) (2.4985, 30.2951) (2.4941, 30.2841) (2.4897, 30.2731) (2.4854, 30.2621) (2.481, 30.2512) (2.4767, 30.2403) (2.4725, 30.2294) (2.4682, 30.2186) (2.464, 30.2078) (2.4598, 30.197) (2.4557, 30.1862) (2.4515, 30.1755) (2.4474, 30.1648) (2.4433, 30.1541) (2.4393, 30.1435) (2.4353, 30.1329) (2.4313, 30.1223) (2.4273, 30.1118) (2.4234, 30.1012) (2.4194, 30.0907) (2.4156, 30.0803) (2.4117, 30.0699) (2.4079, 30.0595) (2.4041, 30.0491) (2.4003, 30.0388) (2.3965, 30.0284) (2.3928, 30.0182) (2.3891, 30.0079) (2.3855, 29.9977) (2.3818, 29.9875) (2.3782, 29.9774) (2.3746, 29.9673) (2.3711, 29.9572) (2.3675, 29.9471) (2.364, 29.9371) (2.3606, 29.9271) (2.3571, 29.9172) (2.3537, 29.9073) (2.3503, 29.8974) (2.3469, 29.8875) (2.3436, 29.8777) (2.3403, 29.868) (2.337, 29.8582) (2.3337, 29.8485) (2.3305, 29.8388) (2.3273, 29.8292) (2.3241, 29.8196) (2.321, 29.81) (2.3178, 29.8005) (2.3147, 29.791) (2.3117, 29.7815) (2.3086, 29.7721) (2.3056, 29.7627) (2.3026, 29.7534) (2.2996, 29.7441) (2.2967, 29.7348) (2.2938, 29.7255) (2.2909, 29.7163) (2.288, 29.7072) (2.2852, 29.6981) (2.2824, 29.689) (2.2796, 29.6799) (2.2769, 29.6709) (2.2741, 29.6619) (2.2714, 29.653) (2.2688, 29.6441) (2.2661, 29.6353) (2.2635, 29.6265) (2.2609, 29.6177) (2.2583, 29.609) (2.2558, 29.6003) (2.2533, 29.5917) (2.2508, 29.583) (2.2483, 29.5745) (2.2458, 29.566) (2.2434, 29.5575) (2.241, 29.5491) (2.2387, 29.5407) (2.2363, 29.5323) (2.234, 29.524) (2.2317, 29.5158) (2.2295, 29.5075) (2.2272, 29.4994) (2.225, 29.4912) (2.2228, 29.4832) (2.2207, 29.4751) (2.2185, 29.4671) (2.2164, 29.4592) (2.2143, 29.4513) (2.2123, 29.4434) (2.2102, 29.4356) (2.2082, 29.4279) (2.2062, 29.4202) (2.2043, 29.4125) (2.2023, 29.4049) (2.2004, 29.3973) (2.1985, 29.3898) (2.1967, 29.3823) (2.1948, 29.3749) (2.193, 29.3675) (2.1912, 29.3602) (2.1895, 29.3529) (2.1877, 29.3457) (2.186, 29.3386) (2.1843, 29.3314) (2.1827, 29.3244) (2.181, 29.3174) (2.1794, 29.3104) (2.1778, 29.3035) (2.1762, 29.2967) (2.1747, 29.2899) (2.1731, 29.2831) (2.1716, 29.2764) (2.1702, 29.2698) (2.1687, 29.2632) (2.1673, 29.2567) (2.1659, 29.2502) (2.1645, 29.2438) (2.1631, 29.2374) (2.1618, 29.2311) (2.1605, 29.2249) (2.1592, 29.2187) (2.1579, 29.2126) (2.1567, 29.2065) (2.1554, 29.2005) (2.1542, 29.1946) (2.153, 29.1887) (2.1519, 29.1829) (2.1507, 29.1771) (2.1496, 29.1714) (2.1485, 29.1658) (2.1475, 29.1602) (2.1464, 29.1547) (2.1454, 29.1493) (2.1444, 29.1439) (2.1434, 29.1386) (2.1424, 29.1334) (2.1415, 29.1282) (2.1406, 29.1231) (2.1397, 29.118) (2.1388, 29.1131) (2.138, 29.1081) (2.1371, 29.1033) (2.1363, 29.0985) (2.1355, 29.0938) (2.1347, 29.0892) (2.134, 29.0847) (2.1332, 29.0802) (2.1325, 29.0758) (2.1318, 29.0714) (2.1312, 29.0672) (2.1305, 29.063) (2.1299, 29.0589) (2.1292, 29.0549) (2.1286, 29.0509) (2.1281, 29.047) (2.1275, 29.0432) (2.127, 29.0395) (2.1264, 29.0359) (2.1259, 29.0323) (2.1254, 29.0289) (2.125, 29.0255) (2.1245, 29.0222) (2.1241, 29.0189) (2.1237, 29.0158) (2.1233, 29.0128) (2.1229, 29.0098) (2.1225, 29.0069) (2.1222, 29.0041) (2.1219, 29.0015) (2.1215, 28.9989) (2.1212, 28.9963) (2.121, 28.9939) (2.1207, 28.9916) (2.1204, 28.9894) (2.1202, 28.9873) (2.12, 28.9852) (2.1198, 28.9833) (2.1196, 28.9815) (2.1194, 28.9798) (2.1192, 28.9781) (2.1191, 28.9766) (2.1189, 28.9752) (2.1188, 28.9739) (2.1187, 28.9727) (2.1186, 28.9716) (2.1185, 28.9706) (2.1184, 28.9698) (2.1184, 28.969) (2.1183, 28.9685) (2.1183, 28.9682) (2.1183, 28.968) (2.1183, 28.9679) knots -1 -1 -1 -1 -1 -1 -0.99583333 -0.99166667 -0.9875 -0.98333333 -0.97916667 -0.975 -0.97083333 -0.96666667 -0.9625 -0.95833333 -0.95416667 -0.95 -0.94583333 -0.94166667 -0.9375 -0.93333333 -0.92916667 -0.925 -0.92083333 -0.91666667 -0.9125 -0.90833333 -0.90416667 -0.9 -0.89583333 -0.89166667 -0.8875 -0.88333333 -0.87916667 -0.875 -0.87083333 -0.86666667 -0.8625 -0.85833333 -0.85416667 -0.85 -0.84583333 -0.84166667 -0.8375 -0.83333333 -0.82916667 -0.825 -0.82083333 -0.81666667 -0.8125 -0.80833333 -0.80416667 -0.8 -0.79583333 -0.79166667 -0.7875 -0.78333333 -0.77916667 -0.775 -0.77083333 -0.76666667 -0.7625 -0.75833333 -0.75416667 -0.75 -0.74583333 -0.74166667 -0.7375 -0.73333333 -0.72916667 -0.725 -0.72083333 -0.71666667 -0.7125 -0.70833333 -0.70416667 -0.7 -0.69583333 -0.69166667 -0.6875 -0.68333333 -0.67916667 -0.675 -0.67083333 -0.66666667 -0.6625 -0.65833333 -0.65416667 -0.65 -0.64583333 -0.64166667 -0.6375 -0.63333333 -0.62916667 -0.625 -0.62083333 -0.61666667 -0.6125 -0.60833333 -0.60416667 -0.6 -0.59583333 -0.59166667 -0.5875 -0.58333333 -0.57916667 -0.575 -0.57083333 -0.56666667 -0.5625 -0.55833333 -0.55416667 -0.55 -0.54583333 -0.54166667 -0.5375 -0.53333333 -0.52916667 -0.525 -0.52083333 -0.51666667 -0.5125 -0.50833333 -0.50416667 -0.5 -0.49583333 -0.49166667 -0.4875 -0.48333333 -0.47916667 -0.475 -0.47083333 -0.46666667 -0.4625 -0.45833333 -0.45416667 -0.45 -0.44583333 -0.44166667 -0.4375 -0.43333333 -0.42916667 -0.425 -0.42083333 -0.41666667 -0.4125 -0.40833333 -0.40416667 -0.4 -0.39583333 -0.39166667 -0.3875 -0.38333333 -0.37916667 -0.375 -0.37083333 -0.36666667 -0.3625 -0.35833333 -0.35416667 -0.35 -0.34583333 -0.34166667 -0.3375 -0.33333333 -0.32916667 -0.325 -0.32083333 -0.31666667 -0.3125 -0.30833333 -0.30416667 -0.3 -0.29583333 -0.29166667 -0.2875 -0.28333333 -0.27916667 -0.275 -0.27083333 -0.26666667 -0.2625 -0.25833333 -0.25416667 -0.25 -0.24583333 -0.24166667 -0.2375 -0.23333333 -0.22916667 -0.225 -0.22083333 -0.21666667 -0.2125 -0.20833333 -0.20416667 -0.2 -0.19583333 -0.19166667 -0.1875 -0.18333333 -0.17916667 -0.175 -0.17083333 -0.16666667 -0.1625 -0.15833333 -0.15416667 -0.15 -0.14583333 -0.14166667 -0.1375 -0.13333333 -0.12916667 -0.125 -0.12083333 -0.11666667 -0.1125 -0.10833333 -0.10416667 -0.1 -0.09583333 -0.09166667 -0.0875 -0.08333333 -0.07916667 -0.075 -0.07083333 -0.06666667 -0.0625 -0.05833333 -0.05416667 -0.05 -0.04583333 -0.04166667 -0.0375 -0.03333333 -0.02916667 -0.025 -0.02083333 -0.01666667 -0.0125 -0.00833333 -0.00416667 0 0 0 0 0 0
  arc A118 (0.4876, 30.9962) -> (-0.4876, 30.9962) centre (0, 0) ccw